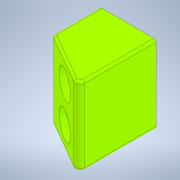
# Autodesk Inventor part: ProximaCustomCaseFront
Saved by Autodesk Inventor 2021 (Build 250183000, 183)
## iProperties
Created: 2022-04-13
Part Number: ProximaCustomCaseFront
Material: Generic
Document SubType Name: Modeling
Designer: ermoz
Density: 1 g/cm^3
Appearance: Default
Author: ermoz
Autodesk Inventor part; units mm, degrees
ref_plane "YZ Plane" through (0, 0, 0) normal (1, 0, 0) x (0, 1, 0)
ref_plane "XZ Plane" through (0, 0, 0) normal (0, 1, 0) x (-1, 0, 0)
ref_plane "XY Plane" through (0, 0, 0) normal (0, 0, 1) x (1, 0, 0)
sketch "Sketch1" plane through (0, 0, 0) normal (0, 1, 0) x (-1, 0, 0)
  line L0 (0, 0) -> (12, 0)
  line L1 (12, 0) -> (12, -10)
  line L2 (12, -10) -> (0, -10)
  line L3 (0, -10) -> (0, 0)
  line L4 (12, 0) -> (0, 6.9282)
  line L5 (12, 0) -> (25.8564, 0) construction
  line L6 (0, 6.9282) -> (0, 0)
  dimension "d0" = 10
  dimension "d1" = 12
  dimension "d2" = 150
  constraints: 14 end point, 2 horizontal, 2 parallel, 1 equal length, 1 perpendicular, 1 vertical
  measures "d0" distance of L0.end L1.end
  measures "d1" distance of L1.end L2.end
  measures "d2" angle of L5 L4
extrude "Extrusion1" add sketch "Sketch1" along normal blind 16.5
sketch "Sketch2" plane through (0, 0, -10) normal (0, 0, -1) x (-1, 0, 0)
  circle A0 centre (6, 4.5) radius 2.8
  circle A1 centre (6, 12) radius 2.8
  line L0 (0, 0) -> (0, 16.5) projected
  line L1 (0, 0) -> (12, 0) projected
  line L2 (0, 16.5) -> (12, 16.5) projected
  dimension "d5" = 5.6
  dimension "d6" = 6
  dimension "d7" = 4.5
  dimension "d8" = 4.5
  constraints: 2 centre point, 1 equal radius, 1 vertical alignment
  measures "d5" diameter of A0
  measures "d6" distance from line of L0 A0.centre
  measures "d7" distance from line of L1 A0.centre
  measures "d8" distance from line of L2 A1.centre
extrude "Extrusion2" cut sketch "Sketch2" against normal through all
fillet "Fillet1" radius 1 2 edges at (0, 8.25, 6.9282) (-12, 8.25, 0)
sketch "Sketch3" plane through (0, 0, -10) normal (0, 0, -1) x (-1, 0, 0)
  circle A0 centre (6, 12) radius 2.8 projected
  circle A1 centre (6, 4.5) radius 2.8 projected
  line L0 (0, 0) -> (12, 0) projected
  line L1 (12, 0) -> (12, 16.5) projected
  line L2 (0, 16.5) -> (12, 16.5) projected
  line L3 (0, 0) -> (0, 16.5) projected
  line L4 (11, 15.5) -> (11, 1)
  line L5 (11, 1) -> (1, 1)
  line L6 (1, 1) -> (1, 15.5)
  line L7 (1, 15.5) -> (11, 15.5)
  dimension "d12" = 1
  constraints: 8 end point, 3 other
  measures "d12" distance between parallel lines of L1 L4
extrude "Extrusion3" cut sketch "Sketch3" against normal blind 3 contours L4 L5 L6 L7
fillet "Fillet2" radius 0.5 14 edges at (-0.5, 16.5, 6.0622) (-6.5, 16.5, 3.1754) (-11.866, 16.5, -0.0774) (-12, 16.5, -5.2887) (0, 16.5, -2.4019) (-0.5, 0, 6.0622) (0, 0, -2.4019) (-11.866, 0, -0.0774) (-12, 0, -5.2887) (-6.5, 0, 3.1754) (-1, 15.5, -8.5) (-11, 15.5, -8.5) (-11, 1, -8.5) (-1, 1, -8.5)
sketch "Sketch4" plane through (0, 0, -7) normal (0, 0, -1) x (-1, 0, 0)
  arc A0 (1, 1.5) -> (1.5, 1) centre (1.5, 1.5) ccw projected
  line L0 (10.5, 1) -> (1.5, 1) projected
  arc A1 (10.5, 1) -> (11, 1.5) centre (10.5, 1.5) ccw projected
  line L1 (11, 15) -> (11, 1.5) projected
  arc A2 (11, 15) -> (10.5, 15.5) centre (10.5, 15) ccw projected
  line L2 (1.5, 15.5) -> (10.5, 15.5) projected
  arc A3 (1.5, 15.5) -> (1, 15) centre (1.5, 15) ccw projected
  line L3 (1, 1.5) -> (1, 15) projected
  circle A4 centre (6, 4.5) radius 2.8 projected
  circle A5 centre (6, 12) radius 2.8 projected
  line L4 (11, 15) -> (11, 1.5) projected
  line L5 (11, 7.75) -> (1, 7.75)
  line L6 (1, 1.5) -> (1, 15) projected
  line L7 (11, 8.75) -> (1, 8.75)
  point P0 (0, 0)
  dimension "d16" = 6.75
  dimension "d17" = 6.75
  constraints: 4 end point, 4 point on line, 2 perpendicular
  measures "d16" distance between parallel lines of L5 L0
  measures "d17" distance between parallel lines of L2 L7
extrude "Extrusion4" cut sketch "Sketch4" against normal blind 7.5 contours L3 L5 L1 A1 L0 A0
extrude "Extrusion5" cut sketch "Sketch4" against normal blind 2 contours L3 A3 L2 A2 L1 L7
equation "\"d8\" = d7"
body "Solid1"
